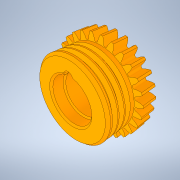
# Autodesk Inventor part: Ролик с шестерней
Saved by Autodesk Inventor 2021.1 (Build 251245010, 245A)
## iProperties
Created: 2026-05-06
Part Number: Ролик с шестерней
Material: Generic
Document SubType Name: Modeling
Designer: Андрей Тарасов
Density: 1 g/cm^3
Appearance: Default
Author: Андрей Тарасов
Autodesk Inventor part; units mm, degrees
(part 1 of 2)
ref_plane "YZ Plane" through (0, 0, 0) normal (1, 0, 0) x (0, 1, 0)
ref_plane "XZ Plane" through (0, 0, 0) normal (0, 1, 0) x (-1, 0, 0)
ref_plane "XY Plane" through (0, 0, 0) normal (0, 0, 1) x (1, 0, 0)
sketch "Sketch1" plane through (0, 0, 0) normal (0, 0, 1) x (1, 0, 0)
  spline S0 degree 3 poles (-1.3158, 14.9422) (-1.2845, 14.8949) (-1.2221, 14.8002) (-1.133, 14.6553) (-1.0475, 14.5082) (-0.9661, 14.3589) (-0.8891, 14.2072) (-0.8168, 14.0532) (-0.7498, 13.8968) (-0.6887, 13.7381) (-0.6345, 13.5769) (-0.5875, 13.4133) (-0.5594, 13.2743) (-0.5393, 13.1627) (-0.5174, 13.0804) (-0.487, 13.0009) (-0.4477, 12.9252) (-0.4044, 12.8686) (-0.3638, 12.829) (-0.3297, 12.8033) (-0.2928, 12.7821) (-0.2536, 12.7654) (-0.2125, 12.7537) (-0.1276, 12.7461) (0, 12.7531) (0.1276, 12.7461) (0.2125, 12.7537) (0.2536, 12.7654) (0.2928, 12.7821) (0.3297, 12.8033) (0.3638, 12.829) (0.4044, 12.8686) (0.4477, 12.9252) (0.487, 13.0009) (0.5174, 13.0804) (0.5393, 13.1627) (0.5594, 13.2743) (0.5875, 13.4133) (0.6345, 13.5769) (0.6887, 13.7381) (0.7498, 13.8968) (0.8168, 14.0532) (0.8891, 14.2072) (0.9661, 14.3589) (1.0475, 14.5082) (1.133, 14.6553) (1.2221, 14.8002) (1.2845, 14.8949) (1.3158, 14.9422) knots 0 0 0 0 0.017008 0.034017 0.051025 0.068033 0.085041 0.10205 0.119057 0.136065 0.153073 0.170079 0.187084 0.195586 0.204089 0.21259 0.221086 0.229576 0.233829 0.238082 0.242331 0.24658 0.250832 0.25508 0.272086 0.289092 0.293339 0.297592 0.30184 0.306089 0.310343 0.314596 0.323086 0.331582 0.340083 0.348586 0.357088 0.374092 0.391099 0.408107 0.425114 0.442122 0.45913 0.476139 0.493147 0.510155 0.527163 0.544172 0.544172 0.544172 0.544172
  circle A0 centre (0, 0) radius 12.75 construction
  circle A1 centre (0, 0) radius 13.1557 construction
  circle A2 centre (0, 0) radius 14 construction
  circle A3 centre (0, 0) radius 15
  spline S1 degree 3 poles (-4.6077, 14.2748) (-4.5668, 14.2356) (-4.4848, 14.1572) (-4.3657, 14.0357) (-4.2496, 13.9114) (-4.137, 13.7839) (-4.0282, 13.6532) (-3.9235, 13.5191) (-3.8234, 13.3816) (-3.7284, 13.2404) (-3.6397, 13.0953) (-3.5575, 12.9462) (-3.4991, 12.817) (-3.4547, 12.7127) (-3.4151, 12.6373) (-3.3677, 12.5665) (-3.3126, 12.5016) (-3.2578, 12.456) (-3.2094, 12.4264) (-3.1705, 12.4089) (-3.1297, 12.3964) (-3.0878, 12.3889) (-3.0452, 12.3867) (-2.9606, 12.3981) (-2.8378, 12.4334) (-2.7119, 12.4549) (-2.6308, 12.4813) (-2.5933, 12.5018) (-2.5588, 12.5267) (-2.5276, 12.5557) (-2.5001, 12.5883) (-2.4693, 12.636) (-2.4397, 12.7008) (-2.4182, 12.7833) (-2.4062, 12.8676) (-2.4032, 12.9527) (-2.4085, 13.0659) (-2.412, 13.2077) (-2.4026, 13.3776) (-2.3856, 13.5469) (-2.3613, 13.7153) (-2.3308, 13.8826) (-2.2946, 14.0488) (-2.2533, 14.2139) (-2.2071, 14.3776) (-2.1565, 14.54) (-2.1019, 14.7011) (-2.0621, 14.8073) (-2.0422, 14.8603) knots 0 0 0 0 0.017008 0.034017 0.051025 0.068033 0.085041 0.10205 0.119057 0.136065 0.153073 0.170079 0.187084 0.195586 0.204089 0.21259 0.221086 0.229576 0.233829 0.238082 0.242331 0.24658 0.250832 0.25508 0.272086 0.289092 0.293339 0.297592 0.30184 0.306089 0.310343 0.314596 0.323086 0.331582 0.340083 0.348586 0.357088 0.374092 0.391099 0.408107 0.425114 0.442122 0.45913 0.476139 0.493147 0.510155 0.527163 0.544172 0.544172 0.544172 0.544172
  spline S2 degree 3 poles (-7.6686, 12.8915) (-7.62, 12.8625) (-7.5226, 12.8043) (-7.3795, 12.7123) (-7.2387, 12.617) (-7.1005, 12.5177) (-6.9653, 12.4145) (-6.8334, 12.3071) (-6.7052, 12.1953) (-6.5812, 12.0788) (-6.4624, 11.957) (-6.3491, 11.83) (-6.2635, 11.717) (-6.1969, 11.6252) (-6.1416, 11.5605) (-6.0796, 11.5021) (-6.0114, 11.451) (-5.9478, 11.4188) (-5.894, 11.4007) (-5.8522, 11.3923) (-5.8097, 11.3892) (-5.7672, 11.3912) (-5.7251, 11.3985) (-5.6453, 11.4285) (-5.5334, 11.4902) (-5.4154, 11.5392) (-5.3422, 11.5829) (-5.3102, 11.6113) (-5.2821, 11.6433) (-5.2581, 11.6785) (-5.2385, 11.7163) (-5.2191, 11.7697) (-5.2047, 11.8395) (-5.2021, 11.9247) (-5.2092, 12.0095) (-5.2252, 12.0932) (-5.2555, 12.2024) (-5.2905, 12.3398) (-5.3192, 12.5076) (-5.3403, 12.6764) (-5.3541, 12.846) (-5.3616, 13.0159) (-5.3633, 13.186) (-5.3597, 13.3561) (-5.3511, 13.526) (-5.3379, 13.6956) (-5.3205, 13.8648) (-5.3053, 13.9771) (-5.2977, 14.0333) knots 0 0 0 0 0.017008 0.034017 0.051025 0.068033 0.085041 0.10205 0.119057 0.136065 0.153073 0.170079 0.187084 0.195586 0.204089 0.21259 0.221086 0.229576 0.233829 0.238082 0.242331 0.24658 0.250832 0.25508 0.272086 0.289092 0.293339 0.297592 0.30184 0.306089 0.310343 0.314596 0.323086 0.331582 0.340083 0.348586 0.357088 0.374092 0.391099 0.408107 0.425114 0.442122 0.45913 0.476139 0.493147 0.510155 0.527163 0.544172 0.544172 0.544172 0.544172
  spline S3 degree 3 poles (-10.345, 10.8619) (-10.2911, 10.8444) (-10.1832, 10.8093) (-10.0233, 10.7515) (-9.8647, 10.6899) (-9.7079, 10.6239) (-9.5532, 10.5533) (-9.4006, 10.478) (-9.2508, 10.3975) (-9.104, 10.3115) (-8.9611, 10.2192) (-8.8223, 10.1206) (-8.7137, 10.0295) (-8.6284, 9.9548) (-8.56, 9.904) (-8.4866, 9.8609) (-8.4087, 9.8262) (-8.3396, 9.8089) (-8.2831, 9.8033) (-8.2405, 9.8045) (-8.1984, 9.8109) (-8.1574, 9.8223) (-8.118, 9.8388) (-8.0468, 9.8857) (-7.9515, 9.9708) (-7.8473, 10.0448) (-7.7857, 10.1038) (-7.7608, 10.1385) (-7.7406, 10.176) (-7.725, 10.2156) (-7.7143, 10.2569) (-7.7073, 10.3132) (-7.7088, 10.3845) (-7.7252, 10.4681) (-7.7509, 10.5493) (-7.7852, 10.6272) (-7.8391, 10.727) (-7.9037, 10.8532) (-7.969, 11.0104) (-8.0271, 11.1702) (-8.0783, 11.3325) (-8.1234, 11.4965) (-8.163, 11.662) (-8.1973, 11.8286) (-8.2268, 11.9961) (-8.2516, 12.1644) (-8.2723, 12.3332) (-8.2825, 12.4462) (-8.2876, 12.5026) knots 0 0 0 0 0.017008 0.034017 0.051025 0.068033 0.085041 0.10205 0.119057 0.136065 0.153073 0.170079 0.187084 0.195586 0.204089 0.21259 0.221086 0.229576 0.233829 0.238082 0.242331 0.24658 0.250832 0.25508 0.272086 0.289092 0.293339 0.297592 0.30184 0.306089 0.310343 0.314596 0.323086 0.331582 0.340083 0.348586 0.357088 0.374092 0.391099 0.408107 0.425114 0.442122 0.45913 0.476139 0.493147 0.510155 0.527163 0.544172 0.544172 0.544172 0.544172
  spline S4 degree 3 poles (-12.5026, 8.2876) (-12.4462, 8.2825) (-12.3332, 8.2723) (-12.1644, 8.2516) (-11.9961, 8.2268) (-11.8286, 8.1973) (-11.662, 8.163) (-11.4965, 8.1234) (-11.3325, 8.0783) (-11.1702, 8.0271) (-11.0104, 7.969) (-10.8532, 7.9037) (-10.727, 7.8391) (-10.6272, 7.7852) (-10.5493, 7.7509) (-10.4681, 7.7252) (-10.3845, 7.7088) (-10.3132, 7.7073) (-10.2569, 7.7143) (-10.2156, 7.725) (-10.176, 7.7406) (-10.1385, 7.7608) (-10.1038, 7.7857) (-10.0448, 7.8473) (-9.9708, 7.9515) (-9.8857, 8.0468) (-9.8388, 8.118) (-9.8223, 8.1574) (-9.8109, 8.1984) (-9.8045, 8.2405) (-9.8033, 8.2831) (-9.8089, 8.3396) (-9.8262, 8.4087) (-9.8609, 8.4866) (-9.904, 8.56) (-9.9548, 8.6284) (-10.0295, 8.7137) (-10.1206, 8.8223) (-10.2192, 8.9611) (-10.3115, 9.104) (-10.3975, 9.2508) (-10.478, 9.4006) (-10.5533, 9.5532) (-10.6239, 9.7079) (-10.6899, 9.8647) (-10.7515, 10.0233) (-10.8093, 10.1832) (-10.8444, 10.2911) (-10.8619, 10.345) knots 0 0 0 0 0.017008 0.034017 0.051025 0.068033 0.085041 0.10205 0.119057 0.136065 0.153073 0.170079 0.187084 0.195586 0.204089 0.21259 0.221086 0.229576 0.233829 0.238082 0.242331 0.24658 0.250832 0.25508 0.272086 0.289092 0.293339 0.297592 0.30184 0.306089 0.310343 0.314596 0.323086 0.331582 0.340083 0.348586 0.357088 0.374092 0.391099 0.408107 0.425114 0.442122 0.45913 0.476139 0.493147 0.510155 0.527163 0.544172 0.544172 0.544172 0.544172
  spline S5 degree 3 poles (-14.0333, 5.2977) (-13.9771, 5.3053) (-13.8648, 5.3205) (-13.6956, 5.3379) (-13.526, 5.3511) (-13.3561, 5.3597) (-13.186, 5.3633) (-13.0159, 5.3616) (-12.846, 5.3541) (-12.6764, 5.3403) (-12.5076, 5.3192) (-12.3398, 5.2905) (-12.2024, 5.2555) (-12.0932, 5.2252) (-12.0095, 5.2092) (-11.9247, 5.2021) (-11.8395, 5.2047) (-11.7697, 5.2191) (-11.7163, 5.2385) (-11.6785, 5.2581) (-11.6433, 5.2821) (-11.6113, 5.3102) (-11.5829, 5.3422) (-11.5392, 5.4154) (-11.4902, 5.5334) (-11.4285, 5.6453) (-11.3985, 5.7251) (-11.3912, 5.7672) (-11.3892, 5.8097) (-11.3923, 5.8522) (-11.4007, 5.894) (-11.4188, 5.9478) (-11.451, 6.0114) (-11.5021, 6.0796) (-11.5605, 6.1416) (-11.6252, 6.1969) (-11.717, 6.2635) (-11.83, 6.3491) (-11.957, 6.4624) (-12.0788, 6.5812) (-12.1953, 6.7052) (-12.3071, 6.8334) (-12.4145, 6.9653) (-12.5177, 7.1005) (-12.617, 7.2387) (-12.7123, 7.3795) (-12.8043, 7.5226) (-12.8625, 7.62) (-12.8915, 7.6686) knots 0 0 0 0 0.017008 0.034017 0.051025 0.068033 0.085041 0.10205 0.119057 0.136065 0.153073 0.170079 0.187084 0.195586 0.204089 0.21259 0.221086 0.229576 0.233829 0.238082 0.242331 0.24658 0.250832 0.25508 0.272086 0.289092 0.293339 0.297592 0.30184 0.306089 0.310343 0.314596 0.323086 0.331582 0.340083 0.348586 0.357088 0.374092 0.391099 0.408107 0.425114 0.442122 0.45913 0.476139 0.493147 0.510155 0.527163 0.544172 0.544172 0.544172 0.544172
  spline S6 degree 3 poles (-14.8603, 2.0422) (-14.8073, 2.0621) (-14.7011, 2.1019) (-14.54, 2.1565) (-14.3776, 2.2071) (-14.2139, 2.2533) (-14.0488, 2.2946) (-13.8826, 2.3308) (-13.7153, 2.3613) (-13.5469, 2.3856) (-13.3776, 2.4026) (-13.2077, 2.412) (-13.0659, 2.4085) (-12.9527, 2.4032) (-12.8676, 2.4062) (-12.7833, 2.4182) (-12.7008, 2.4397) (-12.636, 2.4693) (-12.5883, 2.5001) (-12.5557, 2.5276) (-12.5267, 2.5588) (-12.5018, 2.5933) (-12.4813, 2.6308) (-12.4549, 2.7119) (-12.4334, 2.8378) (-12.3981, 2.9606) (-12.3867, 3.0452) (-12.3889, 3.0878) (-12.3964, 3.1297) (-12.4089, 3.1705) (-12.4264, 3.2094) (-12.456, 3.2578) (-12.5016, 3.3126) (-12.5665, 3.3677) (-12.6373, 3.4151) (-12.7127, 3.4547) (-12.817, 3.4991) (-12.9462, 3.5575) (-13.0953, 3.6397) (-13.2404, 3.7284) (-13.3816, 3.8234) (-13.5191, 3.9235) (-13.6532, 4.0282) (-13.7839, 4.137) (-13.9114, 4.2496) (-14.0357, 4.3657) (-14.1572, 4.4848) (-14.2356, 4.5668) (-14.2748, 4.6077) knots 0 0 0 0 0.017008 0.034017 0.051025 0.068033 0.085041 0.10205 0.119057 0.136065 0.153073 0.170079 0.187084 0.195586 0.204089 0.21259 0.221086 0.229576 0.233829 0.238082 0.242331 0.24658 0.250832 0.25508 0.272086 0.289092 0.293339 0.297592 0.30184 0.306089 0.310343 0.314596 0.323086 0.331582 0.340083 0.348586 0.357088 0.374092 0.391099 0.408107 0.425114 0.442122 0.45913 0.476139 0.493147 0.510155 0.527163 0.544172 0.544172 0.544172 0.544172
  spline S7 degree 3 poles (-14.9422, -1.3158) (-14.8949, -1.2845) (-14.8002, -1.2221) (-14.6553, -1.133) (-14.5082, -1.0475) (-14.3589, -0.9661) (-14.2072, -0.8891) (-14.0532, -0.8168) (-13.8968, -0.7498) (-13.7381, -0.6887) (-13.5769, -0.6345) (-13.4133, -0.5875) (-13.2743, -0.5594) (-13.1627, -0.5393) (-13.0804, -0.5174) (-13.0009, -0.487) (-12.9252, -0.4477) (-12.8686, -0.4044) (-12.829, -0.3638) (-12.8033, -0.3297) (-12.7821, -0.2928) (-12.7654, -0.2536) (-12.7537, -0.2125) (-12.7461, -0.1276) (-12.7531, 0) (-12.7461, 0.1276) (-12.7537, 0.2125) (-12.7654, 0.2536) (-12.7821, 0.2928) (-12.8033, 0.3297) (-12.829, 0.3638) (-12.8686, 0.4044) (-12.9252, 0.4477) (-13.0009, 0.487) (-13.0804, 0.5174) (-13.1627, 0.5393) (-13.2743, 0.5594) (-13.4133, 0.5875) (-13.5769, 0.6345) (-13.7381, 0.6887) (-13.8968, 0.7498) (-14.0532, 0.8168) (-14.2072, 0.8891) (-14.3589, 0.9661) (-14.5082, 1.0475) (-14.6553, 1.133) (-14.8002, 1.2221) (-14.8949, 1.2845) (-14.9422, 1.3158) knots 0 0 0 0 0.017008 0.034017 0.051025 0.068033 0.085041 0.10205 0.119057 0.136065 0.153073 0.170079 0.187084 0.195586 0.204089 0.21259 0.221086 0.229576 0.233829 0.238082 0.242331 0.24658 0.250832 0.25508 0.272086 0.289092 0.293339 0.297592 0.30184 0.306089 0.310343 0.314596 0.323086 0.331582 0.340083 0.348586 0.357088 0.374092 0.391099 0.408107 0.425114 0.442122 0.45913 0.476139 0.493147 0.510155 0.527163 0.544172 0.544172 0.544172 0.544172
  spline S8 degree 3 poles (-14.2748, -4.6077) (-14.2356, -4.5668) (-14.1572, -4.4848) (-14.0357, -4.3657) (-13.9114, -4.2496) (-13.7839, -4.137) (-13.6532, -4.0282) (-13.5191, -3.9235) (-13.3816, -3.8234) (-13.2404, -3.7284) (-13.0953, -3.6397) (-12.9462, -3.5575) (-12.817, -3.4991) (-12.7127, -3.4547) (-12.6373, -3.4151) (-12.5665, -3.3677) (-12.5016, -3.3126) (-12.456, -3.2578) (-12.4264, -3.2094) (-12.4089, -3.1705) (-12.3964, -3.1297) (-12.3889, -3.0878) (-12.3867, -3.0452) (-12.3981, -2.9606) (-12.4334, -2.8378) (-12.4549, -2.7119) (-12.4813, -2.6308) (-12.5018, -2.5933) (-12.5267, -2.5588) (-12.5557, -2.5276) (-12.5883, -2.5001) (-12.636, -2.4693) (-12.7008, -2.4397) (-12.7833, -2.4182) (-12.8676, -2.4062) (-12.9527, -2.4032) (-13.0659, -2.4085) (-13.2077, -2.412) (-13.3776, -2.4026) (-13.5469, -2.3856) (-13.7153, -2.3613) (-13.8826, -2.3308) (-14.0488, -2.2946) (-14.2139, -2.2533) (-14.3776, -2.2071) (-14.54, -2.1565) (-14.7011, -2.1019) (-14.8073, -2.0621) (-14.8603, -2.0422) knots 0 0 0 0 0.017008 0.034017 0.051025 0.068033 0.085041 0.10205 0.119057 0.136065 0.153073 0.170079 0.187084 0.195586 0.204089 0.21259 0.221086 0.229576 0.233829 0.238082 0.242331 0.24658 0.250832 0.25508 0.272086 0.289092 0.293339 0.297592 0.30184 0.306089 0.310343 0.314596 0.323086 0.331582 0.340083 0.348586 0.357088 0.374092 0.391099 0.408107 0.425114 0.442122 0.45913 0.476139 0.493147 0.510155 0.527163 0.544172 0.544172 0.544172 0.544172
  spline S9 degree 3 poles (-12.8915, -7.6686) (-12.8625, -7.62) (-12.8043, -7.5226) (-12.7123, -7.3795) (-12.617, -7.2387) (-12.5177, -7.1005) (-12.4145, -6.9653) (-12.3071, -6.8334) (-12.1953, -6.7052) (-12.0788, -6.5812) (-11.957, -6.4624) (-11.83, -6.3491) (-11.717, -6.2635) (-11.6252, -6.1969) (-11.5605, -6.1416) (-11.5021, -6.0796) (-11.451, -6.0114) (-11.4188, -5.9478) (-11.4007, -5.894) (-11.3923, -5.8522) (-11.3892, -5.8097) (-11.3912, -5.7672) (-11.3985, -5.7251) (-11.4285, -5.6453) (-11.4902, -5.5334) (-11.5392, -5.4154) (-11.5829, -5.3422) (-11.6113, -5.3102) (-11.6433, -5.2821) (-11.6785, -5.2581) (-11.7163, -5.2385) (-11.7697, -5.2191) (-11.8395, -5.2047) (-11.9247, -5.2021) (-12.0095, -5.2092) (-12.0932, -5.2252) (-12.2024, -5.2555) (-12.3398, -5.2905) (-12.5076, -5.3192) (-12.6764, -5.3403) (-12.846, -5.3541) (-13.0159, -5.3616) (-13.186, -5.3633) (-13.3561, -5.3597) (-13.526, -5.3511) (-13.6956, -5.3379) (-13.8648, -5.3205) (-13.9771, -5.3053) (-14.0333, -5.2977) knots 0 0 0 0 0.017008 0.034017 0.051025 0.068033 0.085041 0.10205 0.119057 0.136065 0.153073 0.170079 0.187084 0.195586 0.204089 0.21259 0.221086 0.229576 0.233829 0.238082 0.242331 0.24658 0.250832 0.25508 0.272086 0.289092 0.293339 0.297592 0.30184 0.306089 0.310343 0.314596 0.323086 0.331582 0.340083 0.348586 0.357088 0.374092 0.391099 0.408107 0.425114 0.442122 0.45913 0.476139 0.493147 0.510155 0.527163 0.544172 0.544172 0.544172 0.544172
  spline S10 degree 3 poles (-10.8619, -10.345) (-10.8444, -10.2911) (-10.8093, -10.1832) (-10.7515, -10.0233) (-10.6899, -9.8647) (-10.6239, -9.7079) (-10.5533, -9.5532) (-10.478, -9.4006) (-10.3975, -9.2508) (-10.3115, -9.104) (-10.2192, -8.9611) (-10.1206, -8.8223) (-10.0295, -8.7137) (-9.9548, -8.6284) (-9.904, -8.56) (-9.8609, -8.4866) (-9.8262, -8.4087) (-9.8089, -8.3396) (-9.8033, -8.2831) (-9.8045, -8.2405) (-9.8109, -8.1984) (-9.8223, -8.1574) (-9.8388, -8.118) (-9.8857, -8.0468) (-9.9708, -7.9515) (-10.0448, -7.8473) (-10.1038, -7.7857) (-10.1385, -7.7608) (-10.176, -7.7406) (-10.2156, -7.725) (-10.2569, -7.7143) (-10.3132, -7.7073) (-10.3845, -7.7088) (-10.4681, -7.7252) (-10.5493, -7.7509) (-10.6272, -7.7852) (-10.727, -7.8391) (-10.8532, -7.9037) (-11.0104, -7.969) (-11.1702, -8.0271) (-11.3325, -8.0783) (-11.4965, -8.1234) (-11.662, -8.163) (-11.8286, -8.1973) (-11.9961, -8.2268) (-12.1644, -8.2516) (-12.3332, -8.2723) (-12.4462, -8.2825) (-12.5026, -8.2876) knots 0 0 0 0 0.017008 0.034017 0.051025 0.068033 0.085041 0.10205 0.119057 0.136065 0.153073 0.170079 0.187084 0.195586 0.204089 0.21259 0.221086 0.229576 0.233829 0.238082 0.242331 0.24658 0.250832 0.25508 0.272086 0.289092 0.293339 0.297592 0.30184 0.306089 0.310343 0.314596 0.323086 0.331582 0.340083 0.348586 0.357088 0.374092 0.391099 0.408107 0.425114 0.442122 0.45913 0.476139 0.493147 0.510155 0.527163 0.544172 0.544172 0.544172 0.544172
  spline S11 degree 3 poles (-8.2876, -12.5026) (-8.2825, -12.4462) (-8.2723, -12.3332) (-8.2516, -12.1644) (-8.2268, -11.9961) (-8.1973, -11.8286) (-8.163, -11.662) (-8.1234, -11.4965) (-8.0783, -11.3325) (-8.0271, -11.1702) (-7.969, -11.0104) (-7.9037, -10.8532) (-7.8391, -10.727) (-7.7852, -10.6272) (-7.7509, -10.5493) (-7.7252, -10.4681) (-7.7088, -10.3845) (-7.7073, -10.3132) (-7.7143, -10.2569) (-7.725, -10.2156) (-7.7406, -10.176) (-7.7608, -10.1385) (-7.7857, -10.1038) (-7.8473, -10.0448) (-7.9515, -9.9708) (-8.0468, -9.8857) (-8.118, -9.8388) (-8.1574, -9.8223) (-8.1984, -9.8109) (-8.2405, -9.8045) (-8.2831, -9.8033) (-8.3396, -9.8089) (-8.4087, -9.8262) (-8.4866, -9.8609) (-8.56, -9.904) (-8.6284, -9.9548) (-8.7137, -10.0295) (-8.8223, -10.1206) (-8.9611, -10.2192) (-9.104, -10.3115) (-9.2508, -10.3975) (-9.4006, -10.478) (-9.5532, -10.5533) (-9.7079, -10.6239) (-9.8647, -10.6899) (-10.0233, -10.7515) (-10.1832, -10.8093) (-10.2911, -10.8444) (-10.345, -10.8619) knots 0 0 0 0 0.017008 0.034017 0.051025 0.068033 0.085041 0.10205 0.119057 0.136065 0.153073 0.170079 0.187084 0.195586 0.204089 0.21259 0.221086 0.229576 0.233829 0.238082 0.242331 0.24658 0.250832 0.25508 0.272086 0.289092 0.293339 0.297592 0.30184 0.306089 0.310343 0.314596 0.323086 0.331582 0.340083 0.348586 0.357088 0.374092 0.391099 0.408107 0.425114 0.442122 0.45913 0.476139 0.493147 0.510155 0.527163 0.544172 0.544172 0.544172 0.544172
  spline S12 degree 3 poles (-5.2977, -14.0333) (-5.3053, -13.9771) (-5.3205, -13.8648) (-5.3379, -13.6956) (-5.3511, -13.526) (-5.3597, -13.3561) (-5.3633, -13.186) (-5.3616, -13.0159) (-5.3541, -12.846) (-5.3403, -12.6764) (-5.3192, -12.5076) (-5.2905, -12.3398) (-5.2555, -12.2024) (-5.2252, -12.0932) (-5.2092, -12.0095) (-5.2021, -11.9247) (-5.2047, -11.8395) (-5.2191, -11.7697) (-5.2385, -11.7163) (-5.2581, -11.6785) (-5.2821, -11.6433) (-5.3102, -11.6113) (-5.3422, -11.5829) (-5.4154, -11.5392) (-5.5334, -11.4902) (-5.6453, -11.4285) (-5.7251, -11.3985) (-5.7672, -11.3912) (-5.8097, -11.3892) (-5.8522, -11.3923) (-5.894, -11.4007) (-5.9478, -11.4188) (-6.0114, -11.451) (-6.0796, -11.5021) (-6.1416, -11.5605) (-6.1969, -11.6252) (-6.2635, -11.717) (-6.3491, -11.83) (-6.4624, -11.957) (-6.5812, -12.0788) (-6.7052, -12.1953) (-6.8334, -12.3071) (-6.9653, -12.4145) (-7.1005, -12.5177) (-7.2387, -12.617) (-7.3795, -12.7123) (-7.5226, -12.8043) (-7.62, -12.8625) (-7.6686, -12.8915) knots 0 0 0 0 0.017008 0.034017 0.051025 0.068033 0.085041 0.10205 0.119057 0.136065 0.153073 0.170079 0.187084 0.195586 0.204089 0.21259 0.221086 0.229576 0.233829 0.238082 0.242331 0.24658 0.250832 0.25508 0.272086 0.289092 0.293339 0.297592 0.30184 0.306089 0.310343 0.314596 0.323086 0.331582 0.340083 0.348586 0.357088 0.374092 0.391099 0.408107 0.425114 0.442122 0.45913 0.476139 0.493147 0.510155 0.527163 0.544172 0.544172 0.544172 0.544172
  spline S13 degree 3 poles (-2.0422, -14.8603) (-2.0621, -14.8073) (-2.1019, -14.7011) (-2.1565, -14.54) (-2.2071, -14.3776) (-2.2533, -14.2139) (-2.2946, -14.0488) (-2.3308, -13.8826) (-2.3613, -13.7153) (-2.3856, -13.5469) (-2.4026, -13.3776) (-2.412, -13.2077) (-2.4085, -13.0659) (-2.4032, -12.9527) (-2.4062, -12.8676) (-2.4182, -12.7833) (-2.4397, -12.7008) (-2.4693, -12.636) (-2.5001, -12.5883) (-2.5276, -12.5557) (-2.5588, -12.5267) (-2.5933, -12.5018) (-2.6308, -12.4813) (-2.7119, -12.4549) (-2.8378, -12.4334) (-2.9606, -12.3981) (-3.0452, -12.3867) (-3.0878, -12.3889) (-3.1297, -12.3964) (-3.1705, -12.4089) (-3.2094, -12.4264) (-3.2578, -12.456) (-3.3126, -12.5016) (-3.3677, -12.5665) (-3.4151, -12.6373) (-3.4547, -12.7127) (-3.4991, -12.817) (-3.5575, -12.9462) (-3.6397, -13.0953) (-3.7284, -13.2404) (-3.8234, -13.3816) (-3.9235, -13.5191) (-4.0282, -13.6532) (-4.137, -13.7839) (-4.2496, -13.9114) (-4.3657, -14.0357) (-4.4848, -14.1572) (-4.5668, -14.2356) (-4.6077, -14.2748) knots 0 0 0 0 0.017008 0.034017 0.051025 0.068033 0.085041 0.10205 0.119057 0.136065 0.153073 0.170079 0.187084 0.195586 0.204089 0.21259 0.221086 0.229576 0.233829 0.238082 0.242331 0.24658 0.250832 0.25508 0.272086 0.289092 0.293339 0.297592 0.30184 0.306089 0.310343 0.314596 0.323086 0.331582 0.340083 0.348586 0.357088 0.374092 0.391099 0.408107 0.425114 0.442122 0.45913 0.476139 0.493147 0.510155 0.527163 0.544172 0.544172 0.544172 0.544172
  spline S14 degree 3 poles (1.3158, -14.9422) (1.2845, -14.8949) (1.2221, -14.8002) (1.133, -14.6553) (1.0475, -14.5082) (0.9661, -14.3589) (0.8891, -14.2072) (0.8168, -14.0532) (0.7498, -13.8968) (0.6887, -13.7381) (0.6345, -13.5769) (0.5875, -13.4133) (0.5594, -13.2743) (0.5393, -13.1627) (0.5174, -13.0804) (0.487, -13.0009) (0.4477, -12.9252) (0.4044, -12.8686) (0.3638, -12.829) (0.3297, -12.8033) (0.2928, -12.7821) (0.2536, -12.7654) (0.2125, -12.7537) (0.1276, -12.7461) (0, -12.7531) (-0.1276, -12.7461) (-0.2125, -12.7537) (-0.2536, -12.7654) (-0.2928, -12.7821) (-0.3297, -12.8033) (-0.3638, -12.829) (-0.4044, -12.8686) (-0.4477, -12.9252) (-0.487, -13.0009) (-0.5174, -13.0804) (-0.5393, -13.1627) (-0.5594, -13.2743) (-0.5875, -13.4133) (-0.6345, -13.5769) (-0.6887, -13.7381) (-0.7498, -13.8968) (-0.8168, -14.0532) (-0.8891, -14.2072) (-0.9661, -14.3589) (-1.0475, -14.5082) (-1.133, -14.6553) (-1.2221, -14.8002) (-1.2845, -14.8949) (-1.3158, -14.9422) knots 0 0 0 0 0.017008 0.034017 0.051025 0.068033 0.085041 0.10205 0.119057 0.136065 0.153073 0.170079 0.187084 0.195586 0.204089 0.21259 0.221086 0.229576 0.233829 0.238082 0.242331 0.24658 0.250832 0.25508 0.272086 0.289092 0.293339 0.297592 0.30184 0.306089 0.310343 0.314596 0.323086 0.331582 0.340083 0.348586 0.357088 0.374092 0.391099 0.408107 0.425114 0.442122 0.45913 0.476139 0.493147 0.510155 0.527163 0.544172 0.544172 0.544172 0.544172
  spline S15 degree 3 poles (4.6077, -14.2748) (4.5668, -14.2356) (4.4848, -14.1572) (4.3657, -14.0357) (4.2496, -13.9114) (4.137, -13.7839) (4.0282, -13.6532) (3.9235, -13.5191) (3.8234, -13.3816) (3.7284, -13.2404) (3.6397, -13.0953) (3.5575, -12.9462) (3.4991, -12.817) (3.4547, -12.7127) (3.4151, -12.6373) (3.3677, -12.5665) (3.3126, -12.5016) (3.2578, -12.456) (3.2094, -12.4264) (3.1705, -12.4089) (3.1297, -12.3964) (3.0878, -12.3889) (3.0452, -12.3867) (2.9606, -12.3981) (2.8378, -12.4334) (2.7119, -12.4549) (2.6308, -12.4813) (2.5933, -12.5018) (2.5588, -12.5267) (2.5276, -12.5557) (2.5001, -12.5883) (2.4693, -12.636) (2.4397, -12.7008) (2.4182, -12.7833) (2.4062, -12.8676) (2.4032, -12.9527) (2.4085, -13.0659) (2.412, -13.2077) (2.4026, -13.3776) (2.3856, -13.5469) (2.3613, -13.7153) (2.3308, -13.8826) (2.2946, -14.0488) (2.2533, -14.2139) (2.2071, -14.3776) (2.1565, -14.54) (2.1019, -14.7011) (2.0621, -14.8073) (2.0422, -14.8603) knots 0 0 0 0 0.017008 0.034017 0.051025 0.068033 0.085041 0.10205 0.119057 0.136065 0.153073 0.170079 0.187084 0.195586 0.204089 0.21259 0.221086 0.229576 0.233829 0.238082 0.242331 0.24658 0.250832 0.25508 0.272086 0.289092 0.293339 0.297592 0.30184 0.306089 0.310343 0.314596 0.323086 0.331582 0.340083 0.348586 0.357088 0.374092 0.391099 0.408107 0.425114 0.442122 0.45913 0.476139 0.493147 0.510155 0.527163 0.544172 0.544172 0.544172 0.544172
  spline S16 degree 3 poles (7.6686, -12.8915) (7.62, -12.8625) (7.5226, -12.8043) (7.3795, -12.7123) (7.2387, -12.617) (7.1005, -12.5177) (6.9653, -12.4145) (6.8334, -12.3071) (6.7052, -12.1953) (6.5812, -12.0788) (6.4624, -11.957) (6.3491, -11.83) (6.2635, -11.717) (6.1969, -11.6252) (6.1416, -11.5605) (6.0796, -11.5021) (6.0114, -11.451) (5.9478, -11.4188) (5.894, -11.4007) (5.8522, -11.3923) (5.8097, -11.3892) (5.7672, -11.3912) (5.7251, -11.3985) (5.6453, -11.4285) (5.5334, -11.4902) (5.4154, -11.5392) (5.3422, -11.5829) (5.3102, -11.6113) (5.2821, -11.6433) (5.2581, -11.6785) (5.2385, -11.7163) (5.2191, -11.7697) (5.2047, -11.8395) (5.2021, -11.9247) (5.2092, -12.0095) (5.2252, -12.0932) (5.2555, -12.2024) (5.2905, -12.3398) (5.3192, -12.5076) (5.3403, -12.6764) (5.3541, -12.846) (5.3616, -13.0159) (5.3633, -13.186) (5.3597, -13.3561) (5.3511, -13.526) (5.3379, -13.6956) (5.3205, -13.8648) (5.3053, -13.9771) (5.2977, -14.0333) knots 0 0 0 0 0.017008 0.034017 0.051025 0.068033 0.085041 0.10205 0.119057 0.136065 0.153073 0.170079 0.187084 0.195586 0.204089 0.21259 0.221086 0.229576 0.233829 0.238082 0.242331 0.24658 0.250832 0.25508 0.272086 0.289092 0.293339 0.297592 0.30184 0.306089 0.310343 0.314596 0.323086 0.331582 0.340083 0.348586 0.357088 0.374092 0.391099 0.408107 0.425114 0.442122 0.45913 0.476139 0.493147 0.510155 0.527163 0.544172 0.544172 0.544172 0.544172
  spline S17 degree 3 poles (10.345, -10.8619) (10.2911, -10.8444) (10.1832, -10.8093) (10.0233, -10.7515) (9.8647, -10.6899) (9.7079, -10.6239) (9.5532, -10.5533) (9.4006, -10.478) (9.2508, -10.3975) (9.104, -10.3115) (8.9611, -10.2192) (8.8223, -10.1206) (8.7137, -10.0295) (8.6284, -9.9548) (8.56, -9.904) (8.4866, -9.8609) (8.4087, -9.8262) (8.3396, -9.8089) (8.2831, -9.8033) (8.2405, -9.8045) (8.1984, -9.8109) (8.1574, -9.8223) (8.118, -9.8388) (8.0468, -9.8857) (7.9515, -9.9708) (7.8473, -10.0448) (7.7857, -10.1038) (7.7608, -10.1385) (7.7406, -10.176) (7.725, -10.2156) (7.7143, -10.2569) (7.7073, -10.3132) (7.7088, -10.3845) (7.7252, -10.4681) (7.7509, -10.5493) (7.7852, -10.6272) (7.8391, -10.727) (7.9037, -10.8532) (7.969, -11.0104) (8.0271, -11.1702) (8.0783, -11.3325) (8.1234, -11.4965) (8.163, -11.662) (8.1973, -11.8286) (8.2268, -11.9961) (8.2516, -12.1644) (8.2723, -12.3332) (8.2825, -12.4462) (8.2876, -12.5026) knots 0 0 0 0 0.017008 0.034017 0.051025 0.068033 0.085041 0.10205 0.119057 0.136065 0.153073 0.170079 0.187084 0.195586 0.204089 0.21259 0.221086 0.229576 0.233829 0.238082 0.242331 0.24658 0.250832 0.25508 0.272086 0.289092 0.293339 0.297592 0.30184 0.306089 0.310343 0.314596 0.323086 0.331582 0.340083 0.348586 0.357088 0.374092 0.391099 0.408107 0.425114 0.442122 0.45913 0.476139 0.493147 0.510155 0.527163 0.544172 0.544172 0.544172 0.544172
  spline S18 degree 3 poles (12.5026, -8.2876) (12.4462, -8.2825) (12.3332, -8.2723) (12.1644, -8.2516) (11.9961, -8.2268) (11.8286, -8.1973) (11.662, -8.163) (11.4965, -8.1234) (11.3325, -8.0783) (11.1702, -8.0271) (11.0104, -7.969) (10.8532, -7.9037) (10.727, -7.8391) (10.6272, -7.7852) (10.5493, -7.7509) (10.4681, -7.7252) (10.3845, -7.7088) (10.3132, -7.7073) (10.2569, -7.7143) (10.2156, -7.725) (10.176, -7.7406) (10.1385, -7.7608) (10.1038, -7.7857) (10.0448, -7.8473) (9.9708, -7.9515) (9.8857, -8.0468) (9.8388, -8.118) (9.8223, -8.1574) (9.8109, -8.1984) (9.8045, -8.2405) (9.8033, -8.2831) (9.8089, -8.3396) (9.8262, -8.4087) (9.8609, -8.4866) (9.904, -8.56) (9.9548, -8.6284) (10.0295, -8.7137) (10.1206, -8.8223) (10.2192, -8.9611) (10.3115, -9.104) (10.3975, -9.2508) (10.478, -9.4006) (10.5533, -9.5532) (10.6239, -9.7079) (10.6899, -9.8647) (10.7515, -10.0233) (10.8093, -10.1832) (10.8444, -10.2911) (10.8619, -10.345) knots 0 0 0 0 0.017008 0.034017 0.051025 0.068033 0.085041 0.10205 0.119057 0.136065 0.153073 0.170079 0.187084 0.195586 0.204089 0.21259 0.221086 0.229576 0.233829 0.238082 0.242331 0.24658 0.250832 0.25508 0.272086 0.289092 0.293339 0.297592 0.30184 0.306089 0.310343 0.314596 0.323086 0.331582 0.340083 0.348586 0.357088 0.374092 0.391099 0.408107 0.425114 0.442122 0.45913 0.476139 0.493147 0.510155 0.527163 0.544172 0.544172 0.544172 0.544172
  spline S19 degree 3 poles (14.0333, -5.2977) (13.9771, -5.3053) (13.8648, -5.3205) (13.6956, -5.3379) (13.526, -5.3511) (13.3561, -5.3597) (13.186, -5.3633) (13.0159, -5.3616) (12.846, -5.3541) (12.6764, -5.3403) (12.5076, -5.3192) (12.3398, -5.2905) (12.2024, -5.2555) (12.0932, -5.2252) (12.0095, -5.2092) (11.9247, -5.2021) (11.8395, -5.2047) (11.7697, -5.2191) (11.7163, -5.2385) (11.6785, -5.2581) (11.6433, -5.2821) (11.6113, -5.3102) (11.5829, -5.3422) (11.5392, -5.4154) (11.4902, -5.5334) (11.4285, -5.6453) (11.3985, -5.7251) (11.3912, -5.7672) (11.3892, -5.8097) (11.3923, -5.8522) (11.4007, -5.894) (11.4188, -5.9478) (11.451, -6.0114) (11.5021, -6.0796) (11.5605, -6.1416) (11.6252, -6.1969) (11.717, -6.2635) (11.83, -6.3491) (11.957, -6.4624) (12.0788, -6.5812) (12.1953, -6.7052) (12.3071, -6.8334) (12.4145, -6.9653) (12.5177, -7.1005) (12.617, -7.2387) (12.7123, -7.3795) (12.8043, -7.5226) (12.8625, -7.62) (12.8915, -7.6686) knots 0 0 0 0 0.017008 0.034017 0.051025 0.068033 0.085041 0.10205 0.119057 0.136065 0.153073 0.170079 0.187084 0.195586 0.204089 0.21259 0.221086 0.229576 0.233829 0.238082 0.242331 0.24658 0.250832 0.25508 0.272086 0.289092 0.293339 0.297592 0.30184 0.306089 0.310343 0.314596 0.323086 0.331582 0.340083 0.348586 0.357088 0.374092 0.391099 0.408107 0.425114 0.442122 0.45913 0.476139 0.493147 0.510155 0.527163 0.544172 0.544172 0.544172 0.544172
  spline S20 degree 3 poles (14.8603, -2.0422) (14.8073, -2.0621) (14.7011, -2.1019) (14.54, -2.1565) (14.3776, -2.2071) (14.2139, -2.2533) (14.0488, -2.2946) (13.8826, -2.3308) (13.7153, -2.3613) (13.5469, -2.3856) (13.3776, -2.4026) (13.2077, -2.412) (13.0659, -2.4085) (12.9527, -2.4032) (12.8676, -2.4062) (12.7833, -2.4182) (12.7008, -2.4397) (12.636, -2.4693) (12.5883, -2.5001) (12.5557, -2.5276) (12.5267, -2.5588) (12.5018, -2.5933) (12.4813, -2.6308) (12.4549, -2.7119) (12.4334, -2.8378) (12.3981, -2.9606) (12.3867, -3.0452) (12.3889, -3.0878) (12.3964, -3.1297) (12.4089, -3.1705) (12.4264, -3.2094) (12.456, -3.2578) (12.5016, -3.3126) (12.5665, -3.3677) (12.6373, -3.4151) (12.7127, -3.4547) (12.817, -3.4991) (12.9462, -3.5575) (13.0953, -3.6397) (13.2404, -3.7284) (13.3816, -3.8234) (13.5191, -3.9235) (13.6532, -4.0282) (13.7839, -4.137) (13.9114, -4.2496) (14.0357, -4.3657) (14.1572, -4.4848) (14.2356, -4.5668) (14.2748, -4.6077) knots 0 0 0 0 0.017008 0.034017 0.051025 0.068033 0.085041 0.10205 0.119057 0.136065 0.153073 0.170079 0.187084 0.195586 0.204089 0.21259 0.221086 0.229576 0.233829 0.238082 0.242331 0.24658 0.250832 0.25508 0.272086 0.289092 0.293339 0.297592 0.30184 0.306089 0.310343 0.314596 0.323086 0.331582 0.340083 0.348586 0.357088 0.374092 0.391099 0.408107 0.425114 0.442122 0.45913 0.476139 0.493147 0.510155 0.527163 0.544172 0.544172 0.544172 0.544172
  spline S21 degree 3 poles (14.9422, 1.3158) (14.8949, 1.2845) (14.8002, 1.2221) (14.6553, 1.133) (14.5082, 1.0475) (14.3589, 0.9661) (14.2072, 0.8891) (14.0532, 0.8168) (13.8968, 0.7498) (13.7381, 0.6887) (13.5769, 0.6345) (13.4133, 0.5875) (13.2743, 0.5594) (13.1627, 0.5393) (13.0804, 0.5174) (13.0009, 0.487) (12.9252, 0.4477) (12.8686, 0.4044) (12.829, 0.3638) (12.8033, 0.3297) (12.7821, 0.2928) (12.7654, 0.2536) (12.7537, 0.2125) (12.7461, 0.1276) (12.7531, 0) (12.7461, -0.1276) (12.7537, -0.2125) (12.7654, -0.2536) (12.7821, -0.2928) (12.8033, -0.3297) (12.829, -0.3638) (12.8686, -0.4044) (12.9252, -0.4477) (13.0009, -0.487) (13.0804, -0.5174) (13.1627, -0.5393) (13.2743, -0.5594) (13.4133, -0.5875) (13.5769, -0.6345) (13.7381, -0.6887) (13.8968, -0.7498) (14.0532, -0.8168) (14.2072, -0.8891) (14.3589, -0.9661) (14.5082, -1.0475) (14.6553, -1.133) (14.8002, -1.2221) (14.8949, -1.2845) (14.9422, -1.3158) knots 0 0 0 0 0.017008 0.034017 0.051025 0.068033 0.085041 0.10205 0.119057 0.136065 0.153073 0.170079 0.187084 0.195586 0.204089 0.21259 0.221086 0.229576 0.233829 0.238082 0.242331 0.24658 0.250832 0.25508 0.272086 0.289092 0.293339 0.297592 0.30184 0.306089 0.310343 0.314596 0.323086 0.331582 0.340083 0.348586 0.357088 0.374092 0.391099 0.408107 0.425114 0.442122 0.45913 0.476139 0.493147 0.510155 0.527163 0.544172 0.544172 0.544172 0.544172
  spline S22 degree 3 poles (14.2748, 4.6077) (14.2356, 4.5668) (14.1572, 4.4848) (14.0357, 4.3657) (13.9114, 4.2496) (13.7839, 4.137) (13.6532, 4.0282) (13.5191, 3.9235) (13.3816, 3.8234) (13.2404, 3.7284) (13.0953, 3.6397) (12.9462, 3.5575) (12.817, 3.4991) (12.7127, 3.4547) (12.6373, 3.4151) (12.5665, 3.3677) (12.5016, 3.3126) (12.456, 3.2578) (12.4264, 3.2094) (12.4089, 3.1705) (12.3964, 3.1297) (12.3889, 3.0878) (12.3867, 3.0452) (12.3981, 2.9606) (12.4334, 2.8378) (12.4549, 2.7119) (12.4813, 2.6308) (12.5018, 2.5933) (12.5267, 2.5588) (12.5557, 2.5276) (12.5883, 2.5001) (12.636, 2.4693) (12.7008, 2.4397) (12.7833, 2.4182) (12.8676, 2.4062) (12.9527, 2.4032) (13.0659, 2.4085) (13.2077, 2.412) (13.3776, 2.4026) (13.5469, 2.3856) (13.7153, 2.3613) (13.8826, 2.3308) (14.0488, 2.2946) (14.2139, 2.2533) (14.3776, 2.2071) (14.54, 2.1565) (14.7011, 2.1019) (14.8073, 2.0621) (14.8603, 2.0422) knots 0 0 0 0 0.017008 0.034017 0.051025 0.068033 0.085041 0.10205 0.119057 0.136065 0.153073 0.170079 0.187084 0.195586 0.204089 0.21259 0.221086 0.229576 0.233829 0.238082 0.242331 0.24658 0.250832 0.25508 0.272086 0.289092 0.293339 0.297592 0.30184 0.306089 0.310343 0.314596 0.323086 0.331582 0.340083 0.348586 0.357088 0.374092 0.391099 0.408107 0.425114 0.442122 0.45913 0.476139 0.493147 0.510155 0.527163 0.544172 0.544172 0.544172 0.544172
  spline S23 degree 3 poles (12.8915, 7.6686) (12.8625, 7.62) (12.8043, 7.5226) (12.7123, 7.3795) (12.617, 7.2387) (12.5177, 7.1005) (12.4145, 6.9653) (12.3071, 6.8334) (12.1953, 6.7052) (12.0788, 6.5812) (11.957, 6.4624) (11.83, 6.3491) (11.717, 6.2635) (11.6252, 6.1969) (11.5605, 6.1416) (11.5021, 6.0796) (11.451, 6.0114) (11.4188, 5.9478) (11.4007, 5.894) (11.3923, 5.8522) (11.3892, 5.8097) (11.3912, 5.7672) (11.3985, 5.7251) (11.4285, 5.6453) (11.4902, 5.5334) (11.5392, 5.4154) (11.5829, 5.3422) (11.6113, 5.3102) (11.6433, 5.2821) (11.6785, 5.2581) (11.7163, 5.2385) (11.7697, 5.2191) (11.8395, 5.2047) (11.9247, 5.2021) (12.0095, 5.2092) (12.0932, 5.2252) (12.2024, 5.2555) (12.3398, 5.2905) (12.5076, 5.3192) (12.6764, 5.3403) (12.846, 5.3541) (13.0159, 5.3616) (13.186, 5.3633) (13.3561, 5.3597) (13.526, 5.3511) (13.6956, 5.3379) (13.8648, 5.3205) (13.9771, 5.3053) (14.0333, 5.2977) knots 0 0 0 0 0.017008 0.034017 0.051025 0.068033 0.085041 0.10205 0.119057 0.136065 0.153073 0.170079 0.187084 0.195586 0.204089 0.21259 0.221086 0.229576 0.233829 0.238082 0.242331 0.24658 0.250832 0.25508 0.272086 0.289092 0.293339 0.297592 0.30184 0.306089 0.310343 0.314596 0.323086 0.331582 0.340083 0.348586 0.357088 0.374092 0.391099 0.408107 0.425114 0.442122 0.45913 0.476139 0.493147 0.510155 0.527163 0.544172 0.544172 0.544172 0.544172
  spline S24 degree 3 poles (10.8619, 10.345) (10.8444, 10.2911) (10.8093, 10.1832) (10.7515, 10.0233) (10.6899, 9.8647) (10.6239, 9.7079) (10.5533, 9.5532) (10.478, 9.4006) (10.3975, 9.2508) (10.3115, 9.104) (10.2192, 8.9611) (10.1206, 8.8223) (10.0295, 8.7137) (9.9548, 8.6284) (9.904, 8.56) (9.8609, 8.4866) (9.8262, 8.4087) (9.8089, 8.3396) (9.8033, 8.2831) (9.8045, 8.2405) (9.8109, 8.1984) (9.8223, 8.1574) (9.8388, 8.118) (9.8857, 8.0468) (9.9708, 7.9515) (10.0448, 7.8473) (10.1038, 7.7857) (10.1385, 7.7608) (10.176, 7.7406) (10.2156, 7.725) (10.2569, 7.7143) (10.3132, 7.7073) (10.3845, 7.7088) (10.4681, 7.7252) (10.5493, 7.7509) (10.6272, 7.7852) (10.727, 7.8391) (10.8532, 7.9037) (11.0104, 7.969) (11.1702, 8.0271) (11.3325, 8.0783) (11.4965, 8.1234) (11.662, 8.163) (11.8286, 8.1973) (11.9961, 8.2268) (12.1644, 8.2516) (12.3332, 8.2723) (12.4462, 8.2825) (12.5026, 8.2876) knots 0 0 0 0 0.017008 0.034017 0.051025 0.068033 0.085041 0.10205 0.119057 0.136065 0.153073 0.170079 0.187084 0.195586 0.204089 0.21259 0.221086 0.229576 0.233829 0.238082 0.242331 0.24658 0.250832 0.25508 0.272086 0.289092 0.293339 0.297592 0.30184 0.306089 0.310343 0.314596 0.323086 0.331582 0.340083 0.348586 0.357088 0.374092 0.391099 0.408107 0.425114 0.442122 0.45913 0.476139 0.493147 0.510155 0.527163 0.544172 0.544172 0.544172 0.544172
  spline S25 degree 3 poles (8.2876, 12.5026) (8.2825, 12.4462) (8.2723, 12.3332) (8.2516, 12.1644) (8.2268, 11.9961) (8.1973, 11.8286) (8.163, 11.662) (8.1234, 11.4965) (8.0783, 11.3325) (8.0271, 11.1702) (7.969, 11.0104) (7.9037, 10.8532) (7.8391, 10.727) (7.7852, 10.6272) (7.7509, 10.5493) (7.7252, 10.4681) (7.7088, 10.3845) (7.7073, 10.3132) (7.7143, 10.2569) (7.725, 10.2156) (7.7406, 10.176) (7.7608, 10.1385) (7.7857, 10.1038) (7.8473, 10.0448) (7.9515, 9.9708) (8.0468, 9.8857) (8.118, 9.8388) (8.1574, 9.8223) (8.1984, 9.8109) (8.2405, 9.8045) (8.2831, 9.8033) (8.3396, 9.8089) (8.4087, 9.8262) (8.4866, 9.8609) (8.56, 9.904) (8.6284, 9.9548) (8.7137, 10.0295) (8.8223, 10.1206) (8.9611, 10.2192) (9.104, 10.3115) (9.2508, 10.3975) (9.4006, 10.478) (9.5532, 10.5533) (9.7079, 10.6239) (9.8647, 10.6899) (10.0233, 10.7515) (10.1832, 10.8093) (10.2911, 10.8444) (10.345, 10.8619) knots 0 0 0 0 0.017008 0.034017 0.051025 0.068033 0.085041 0.10205 0.119057 0.136065 0.153073 0.170079 0.187084 0.195586 0.204089 0.21259 0.221086 0.229576 0.233829 0.238082 0.242331 0.24658 0.250832 0.25508 0.272086 0.289092 0.293339 0.297592 0.30184 0.306089 0.310343 0.314596 0.323086 0.331582 0.340083 0.348586 0.357088 0.374092 0.391099 0.408107 0.425114 0.442122 0.45913 0.476139 0.493147 0.510155 0.527163 0.544172 0.544172 0.544172 0.544172
  spline S26 degree 3 poles (5.2977, 14.0333) (5.3053, 13.9771) (5.3205, 13.8648) (5.3379, 13.6956) (5.3511, 13.526) (5.3597, 13.3561) (5.3633, 13.186) (5.3616, 13.0159) (5.3541, 12.846) (5.3403, 12.6764) (5.3192, 12.5076) (5.2905, 12.3398) (5.2555, 12.2024) (5.2252, 12.0932) (5.2092, 12.0095) (5.2021, 11.9247) (5.2047, 11.8395) (5.2191, 11.7697) (5.2385, 11.7163) (5.2581, 11.6785) (5.2821, 11.6433) (5.3102, 11.6113) (5.3422, 11.5829) (5.4154, 11.5392) (5.5334, 11.4902) (5.6453, 11.4285) (5.7251, 11.3985) (5.7672, 11.3912) (5.8097, 11.3892) (5.8522, 11.3923) (5.894, 11.4007) (5.9478, 11.4188) (6.0114, 11.451) (6.0796, 11.5021) (6.1416, 11.5605) (6.1969, 11.6252) (6.2635, 11.717) (6.3491, 11.83) (6.4624, 11.957) (6.5812, 12.0788) (6.7052, 12.1953) (6.8334, 12.3071) (6.9653, 12.4145) (7.1005, 12.5177) (7.2387, 12.617) (7.3795, 12.7123) (7.5226, 12.8043) (7.62, 12.8625) (7.6686, 12.8915) knots 0 0 0 0 0.017008 0.034017 0.051025 0.068033 0.085041 0.10205 0.119057 0.136065 0.153073 0.170079 0.187084 0.195586 0.204089 0.21259 0.221086 0.229576 0.233829 0.238082 0.242331 0.24658 0.250832 0.25508 0.272086 0.289092 0.293339 0.297592 0.30184 0.306089 0.310343 0.314596 0.323086 0.331582 0.340083 0.348586 0.357088 0.374092 0.391099 0.408107 0.425114 0.442122 0.45913 0.476139 0.493147 0.510155 0.527163 0.544172 0.544172 0.544172 0.544172
  spline S27 degree 3 poles (2.0422, 14.8603) (2.0621, 14.8073) (2.1019, 14.7011) (2.1565, 14.54) (2.2071, 14.3776) (2.2533, 14.2139) (2.2946, 14.0488) (2.3308, 13.8826) (2.3613, 13.7153) (2.3856, 13.5469) (2.4026, 13.3776) (2.412, 13.2077) (2.4085, 13.0659) (2.4032, 12.9527) (2.4062, 12.8676) (2.4182, 12.7833) (2.4397, 12.7008) (2.4693, 12.636) (2.5001, 12.5883) (2.5276, 12.5557) (2.5588, 12.5267) (2.5933, 12.5018) (2.6308, 12.4813) (2.7119, 12.4549) (2.8378, 12.4334) (2.9606, 12.3981) (3.0452, 12.3867) (3.0878, 12.3889) (3.1297, 12.3964) (3.1705, 12.4089) (3.2094, 12.4264) (3.2578, 12.456) (3.3126, 12.5016) (3.3677, 12.5665) (3.4151, 12.6373) (3.4547, 12.7127) (3.4991, 12.817) (3.5575, 12.9462) (3.6397, 13.0953) (3.7284, 13.2404) (3.8234, 13.3816) (3.9235, 13.5191) (4.0282, 13.6532) (4.137, 13.7839) (4.2496, 13.9114) (4.3657, 14.0357) (4.4848, 14.1572) (4.5668, 14.2356) (4.6077, 14.2748) knots 0 0 0 0 0.017008 0.034017 0.051025 0.068033 0.085041 0.10205 0.119057 0.136065 0.153073 0.170079 0.187084 0.195586 0.204089 0.21259 0.221086 0.229576 0.233829 0.238082 0.242331 0.24658 0.250832 0.25508 0.272086 0.289092 0.293339 0.297592 0.30184 0.306089 0.310343 0.314596 0.323086 0.331582 0.340083 0.348586 0.357088 0.374092 0.391099 0.408107 0.425114 0.442122 0.45913 0.476139 0.493147 0.510155 0.527163 0.544172 0.544172 0.544172 0.544172
  circle A4 centre (0, 0) radius 7
  point P0 (-1.2229, 14.7997)
  point P1 (-1.1336, 14.6549)
  point P2 (-1.0482, 14.5079)
  point P3 (-0.9668, 14.3585)
  point P4 (-0.8899, 14.2068)
  point P5 (-0.8177, 14.0528)
  point P6 (-0.7508, 13.8965)
  point P7 (-0.6898, 13.7377)
  point P8 (-0.6357, 13.5765)
  point P9 (-0.5897, 13.4127)
  point P10 (-0.5545, 13.2464)
  point P11 (-0.5381, 13.1629)
  point P12 (-0.516, 13.0808)
  point P13 (-0.4855, 13.0015)
  point P14 (-0.4455, 12.9265)
  point P15 (-0.3938, 12.8592)
  point P16 (-0.3632, 12.8297)
  point P17 (-0.3292, 12.804)
  point P18 (-0.2924, 12.7828)
  point P19 (-0.2533, 12.7662)
  point P20 (-0.2123, 12.755)
  point P21 (-0.1701, 12.7503)
  point P22 (0, 12.75)
  point P23 (0.1701, 12.7503)
  point P24 (0.2123, 12.755)
  point P25 (0.2533, 12.7662)
  point P26 (0.2924, 12.7828)
  point P27 (0.3292, 12.804)
  point P28 (0.3632, 12.8297)
  point P29 (0.3938, 12.8592)
  point P30 (0.4455, 12.9265)
  point P31 (0.4855, 13.0015)
  point P32 (0.516, 13.0808)
  point P33 (0.5381, 13.1629)
  point P34 (0.5545, 13.2464)
  point P35 (0.5897, 13.4127)
  point P36 (0.6357, 13.5765)
  point P37 (0.6898, 13.7377)
  point P38 (0.7508, 13.8965)
  point P39 (0.8177, 14.0528)
  point P40 (0.8899, 14.2068)
  point P41 (0.9668, 14.3585)
  point P42 (1.0482, 14.5079)
  point P43 (1.1336, 14.6549)
  point P44 (1.2229, 14.7997)
  point P45 (-4.4854, 14.1566)
  point P46 (-4.3662, 14.0352)
  point P47 (-4.2502, 13.9109)
  point P48 (-4.1377, 13.7834)
  point P49 (-4.0289, 13.6526)
  point P50 (-3.9242, 13.5185)
  point P51 (-3.8242, 13.381)
  point P52 (-3.7294, 13.2397)
  point P53 (-3.6408, 13.0946)
  point P54 (-3.5595, 12.9452)
  point P55 (-3.4882, 12.7908)
  point P56 (-3.4537, 12.7132)
  point P57 (-3.4138, 12.638)
  point P58 (-3.3664, 12.5675)
  point P59 (-3.3108, 12.5033)
  point P60 (-3.2453, 12.4492)
  point P61 (-3.2089, 12.4272)
  point P62 (-3.1701, 12.4098)
  point P63 (-3.1295, 12.3973)
  point P64 (-3.0877, 12.3898)
  point P65 (-3.0452, 12.388)
  point P66 (-2.8371, 12.4303)
  point P67 (-2.6714, 12.4685)
  point P68 (-3.003, 12.3928)
  point P69 (-2.5938, 12.5025)
  point P70 (-2.5594, 12.5274)
  point P71 (-2.5282, 12.5563)
  point P72 (-2.5008, 12.5888)
  point P73 (-2.4775, 12.6244)
  point P74 (-2.442, 12.7015)
  point P75 (-2.4198, 12.7835)
  point P76 (-2.4044, 12.9526)
  point P77 (-2.407, 13.0376)
  point P78 (-2.4097, 13.2077)
  point P79 (-2.4013, 13.3775)
  point P80 (-2.3844, 13.5467)
  point P81 (-2.3603, 13.7151)
  point P82 (-2.3299, 13.8824)
  point P83 (-2.2938, 14.0486)
  point P84 (-2.2525, 14.2136)
  point P85 (-2.2064, 14.3774)
  point P86 (-2.1558, 14.5398)
  point P87 (-2.1011, 14.7008)
  point P88 (-2.6313, 12.4825)
  point P89 (-2.4077, 12.8677)
  point P90 (-7.5231, 12.8035)
  point P91 (-7.3799, 12.7118)
  point P92 (-7.2391, 12.6163)
  point P93 (-7.101, 12.5171)
  point P94 (-6.9658, 12.4138)
  point P95 (-6.834, 12.3064)
  point P96 (-6.7059, 12.1945)
  point P97 (-6.5821, 12.0779)
  point P98 (-6.4633, 11.9562)
  point P99 (-6.3508, 11.8286)
  point P100 (-6.247, 11.6939)
  point P101 (-6.196, 11.6259)
  point P102 (-6.1405, 11.5615)
  point P103 (-6.0785, 11.5033)
  point P104 (-6.01, 11.4531)
  point P105 (-5.9342, 11.4149)
  point P106 (-5.8938, 11.4016)
  point P107 (-5.8521, 11.3932)
  point P108 (-5.8097, 11.3901)
  point P109 (-5.7673, 11.3921)
  point P110 (-5.7255, 11.3998)
  point P111 (-5.532, 11.4874)
  point P112 (-5.3789, 11.5614)
  point P113 (-5.6854, 11.4138)
  point P114 (-5.3109, 11.6119)
  point P115 (-5.2828, 11.6438)
  point P116 (-5.2589, 11.6789)
  point P117 (-5.2394, 11.7167)
  point P118 (-5.2246, 11.7566)
  point P119 (-5.2072, 11.8397)
  point P120 (-5.2037, 11.9246)
  point P121 (-5.2263, 12.0929)
  point P122 (-5.2478, 12.1752)
  point P123 (-5.2883, 12.3403)
  point P124 (-5.3179, 12.5078)
  point P125 (-5.3391, 12.6765)
  point P126 (-5.353, 12.846)
  point P127 (-5.3606, 13.0159)
  point P128 (-5.3624, 13.186)
  point P129 (-5.3588, 13.356)
  point P130 (-5.3503, 13.5259)
  point P131 (-5.3372, 13.6955)
  point P132 (-5.3196, 13.8647)
  point P133 (-5.3429, 11.584)
  point P134 (-5.2107, 12.0093)
  point P135 (-10.1835, 10.8084)
  point P136 (-10.0235, 10.7509)
  point P137 (-9.865, 10.6892)
  point P138 (-9.7083, 10.6231)
  point P139 (-9.5535, 10.5525)
  point P140 (-9.4011, 10.4771)
  point P141 (-9.2513, 10.3966)
  point P142 (-9.1046, 10.3105)
  point P143 (-8.9618, 10.2182)
  point P144 (-8.8237, 10.1188)
  point P145 (-8.6925, 10.0107)
  point P146 (-8.6277, 9.9557)
  point P147 (-8.5592, 9.9053)
  point P148 (-8.4859, 9.8623)
  point P149 (-8.4079, 9.8285)
  point P150 (-8.3254, 9.8082)
  point P151 (-8.2831, 9.8042)
  point P152 (-8.2406, 9.8053)
  point P153 (-8.1986, 9.8117)
  point P154 (-8.1577, 9.8231)
  point P155 (-8.1186, 9.8399)
  point P156 (-7.9495, 9.9684)
  point P157 (-7.8167, 10.0746)
  point P158 (-8.0826, 9.8626)
  point P159 (-7.7616, 10.139)
  point P160 (-7.7414, 10.1763)
  point P161 (-7.7258, 10.2159)
  point P162 (-7.7152, 10.2571)
  point P163 (-7.7097, 10.2992)
  point P164 (-7.7112, 10.3841)
  point P165 (-7.7267, 10.4677)
  point P166 (-7.7862, 10.6267)
  point P167 (-7.8254, 10.7022)
  point P168 (-7.9017, 10.8541)
  point P169 (-7.9678, 11.0108)
  point P170 (-8.026, 11.1706)
  point P171 (-8.0773, 11.3328)
  point P172 (-8.1225, 11.4968)
  point P173 (-8.1621, 11.6622)
  point P174 (-8.1965, 11.8287)
  point P175 (-8.226, 11.9962)
  point P176 (-8.2509, 12.1645)
  point P177 (-8.2714, 12.3333)
  point P178 (-7.7867, 10.1046)
  point P179 (-7.7523, 10.5487)
  point P180 (-12.3333, 8.2714)
  point P181 (-12.1645, 8.2509)
  point P182 (-11.9962, 8.226)
  point P183 (-11.8287, 8.1965)
  point P184 (-11.6622, 8.1621)
  point P185 (-11.4968, 8.1225)
  point P186 (-11.3328, 8.0773)
  point P187 (-11.1706, 8.026)
  point P188 (-11.0108, 7.9678)
  point P189 (-10.8541, 7.9017)
  point P190 (-10.7022, 7.8254)
  point P191 (-10.6267, 7.7862)
  point P192 (-10.5487, 7.7523)
  point P193 (-10.4677, 7.7267)
  point P194 (-10.3841, 7.7112)
  point P195 (-10.2992, 7.7097)
  point P196 (-10.2571, 7.7152)
  point P197 (-10.2159, 7.7258)
  point P198 (-10.1763, 7.7414)
  point P199 (-10.139, 7.7616)
  dimension "d4" = 360
  dimension "d6" = 14
  constraints: 4 centre point, 1 coincident, 2716 other
  measures "d6" diameter of A4
extrude "Выдавливание1" add sketch "Sketch1" against normal blind 5 contours S0 A3 S27 S26 S25 S24 S23 S22 S21 S20 S19 S18 S17 S16 S15 S14 S13 S12 S11 S10 S9 S8 S7 S6 S5 S4 S3 S2 S1
sketch "Эскиз2" plane through (0, 0, 0) normal (1, 0, 0) x (0, 1, 0)
  line L0 (0, 9) -> (12.5, 9)
  line L1 (12.5, 9) -> (12.5, 0)
  line L2 (12.5, 0) -> (0, 0)
  line L3 (0, -11.4) -> (0, 33.4) construction
  line L4 (11.5, 9) -> (11.5, 0) construction
  line L5 (11.5, 2.3) -> (12.5, 2.3) construction
  line L6 (-20.9191, 0) -> (20.9191, 0) construction
  arc A0 (11.375, 2.0835) -> (11.375, 2.5165) centre (11.5, 2.3) ccw construction
  line L7 (12.5, 3.166) -> (11.375, 2.5165)
  line L8 (12.5, 1.434) -> (11.375, 2.0835)
  arc A1 (11.375, 2.5165) -> (11.375, 2.0835) centre (11.5, 2.3) ccw
  line L9 (12.5, 5.366) -> (11.375, 4.7165)
  arc A2 (11.375, 4.7165) -> (11.375, 4.2835) centre (11.5, 4.5) ccw
  line L10 (12.5, 3.634) -> (11.375, 4.2835)
  line L11 (12.5, 7.566) -> (11.375, 6.9165)
  arc A3 (11.375, 6.9165) -> (11.375, 6.4835) centre (11.5, 6.7) ccw
  line L12 (12.5, 5.834) -> (11.375, 6.4835)
  line L13 (7, 9) -> (7, -0.5)
  line L14 (7, 4.5) -> (6.5, 4.5)
  line L15 (6.5, 4.5) -> (6.5, -0.5)
  line L16 (6.5, -0.5) -> (7, -0.5)
  point P0 (12.5, 3.634)
  point P1 (7, 0)
  dimension "d7" = 12.5
  dimension "d8" = 9
  dimension "d9" = 2.3
  dimension "d10" = 1
  dimension "d11" = 0.5
  dimension "d12" = 30
  dimension "d13" = 30
  dimension "d16" = 2.2
  dimension "d21" = 7
  dimension "d22" = 0.5
  dimension "d23" = 4.5
  dimension "d24" = 0.5
  constraints: 30 end point, 9 point on line, 8 point on circle, 6 perpendicular, 4 centre point, 2 horizontal, 2 tangent, 2 vertical, 1 coincident, 1 collinear, 16 other
  measures "d7" distance between parallel lines of L1 L3
  measures "d8" distance between parallel lines of L2 L0
  measures "d9" distance between parallel lines of L2 L5
  measures "d10" distance between parallel lines of L4 L1
  measures "d11" diameter of A0
  measures "d12" angle of L5 L7
  measures "d13" angle of L8 L5
  measures "d16" distance of L7.start L9.start
  measures "d21" distance between parallel lines of L3 L13
  measures "d22" distance between parallel lines of L13 L15
  measures "d23" distance between parallel lines of L14 L0
  measures "d24" distance between parallel lines of L2 L16
revolve "Вращение1" add sketch "Эскиз2" angle 360 about axis through (0, 0, -10) along (0, 0, 1) contours L0 L1 L11 A3 L12 L9 A2 L10 L7 A1 L8 L2 L13 | L13 L2 L15 L14 | L13 L16 L15 L2
sketch "Эскиз3" plane through (0, 0, 9) normal (0, 0, 1) x (1, 0, 0)
  line L0 (0, -20.9191) -> (0, 20.9191) construction
  circle A0 centre (0, 0) radius 7 construction
  arc A1 (0.9004, 7.4351) -> (-0.9004, 7.4351) centre (0, 7) ccw
  arc A2 (-1.691, 6.7927) -> (1.691, 6.7927) centre (0, 0) ccw
  arc A3 (-1.691, 6.7927) -> (-0.9004, 7.4351) centre (-1.9809, 7.9571) ccw
  arc A4 (0.9004, 7.4351) -> (1.691, 6.7927) centre (1.9809, 7.9571) ccw
  circle A5 centre (0, 7) radius 1.7037
  point P0 (1.691, 6.7927)
  dimension "d38" = 1
  dimension "d39" = 1.2
  constraints: 8 point on circle, 4 centre point, 4 tangent, 2 coincident, 1 equal radius, 1 point on line, 1 vertical alignment, 5 other
  measures "d38" radius of A1
  measures "d39" radius of A3
extrude "Выдавливание2" cut sketch "Эскиз3" against normal up to surface (14 mm away) contours A4 A5 A3 A1 picked at (0, 6.5739)
chamfer "Фаска1" distance 0.6 angle 45 2 edges at (0, -7, 9) (0, -7, -5)
chamfer "Фаска2" distance 0.8 angle 45 1 edges at (0, -12.5, 9)
feature "Толщина1" [suppressed]